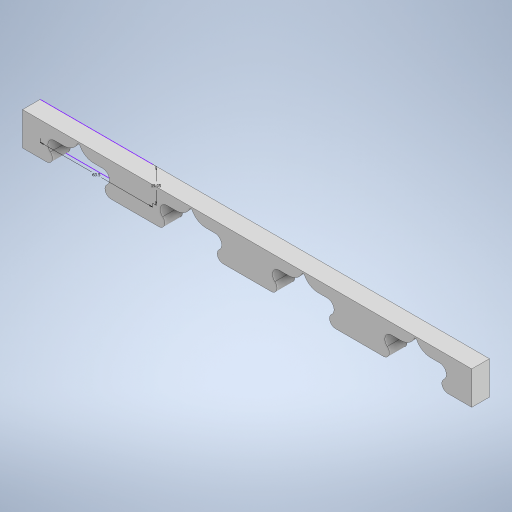
# Autodesk Inventor part: Zipperteethv2
Saved by Autodesk Inventor 2023.1 (Build 271208000, 208)
## iProperties
Created: 2022-09-20
Part Number: Zipperteethv2
Material: Generic
Document SubType Name: Modeling
Designer: Grimm
Density: 1 g/cm^3
Appearance: Default
Author: Grimm
Autodesk Inventor part; units mm, degrees
ref_plane "YZ Plane" through (0, 0, 0) normal (1, 0, 0) x (0, 1, 0)
ref_plane "XZ Plane" through (0, 0, 0) normal (0, 1, 0) x (-1, 0, 0)
ref_plane "XY Plane" through (0, 0, 0) normal (0, 0, 1) x (1, 0, 0)
sketch "Sketch1" plane through (0, 0, 0) normal (0, 0, 1) x (1, 0, 0)
  line L0 (-11.2052, 4.8709) -> (52.2948, 4.8709)
  line L1 (52.2948, 4.8709) -> (52.2948, -14.1791)
  line L2 (52.2948, -14.1791) -> (-11.2052, -14.1791)
  line L3 (-11.2052, -14.1791) -> (-11.2052, 4.8709)
  point P0 (0, 0)
  dimension "d0" = 63.5
  dimension "d1" = 19.05
  constraints: 8 end point, 2 parallel, 1 horizontal, 1 perpendicular
  measures "d0" distance of L1.end L2.end
  measures "d1" distance of L0.end L1.end
extrude "Extrusion1" add sketch "Sketch1" along normal blind 10
sketch "Sketch2" plane through (0, 0, 10) normal (0, 0, 1) x (1, 0, 0)
  line L0 (52.2948, 4.8709) -> (-11.2052, 4.8709) projected
  line L1 (20.5448, 4.8709) -> (20.5448, 2.3309)
  line L2 (-11.2052, -14.1791) -> (52.2948, -14.1791) projected
  arc A0 (7.0053, -1.4791) -> (4.6698, -7.8291) centre (7.0053, -5.0836) ccw
  arc A1 (2.3343, -14.1791) -> (4.6698, -7.8291) centre (2.3343, -10.5746) ccw
  arc A2 (36.4198, -7.8291) -> (34.0843, -1.4791) centre (34.0843, -5.0836) ccw
  arc A3 (36.4198, -7.8291) -> (38.7553, -14.1791) centre (38.7553, -10.5746) ccw
  line L3 (7.0053, -1.4791) -> (34.0843, -1.4791)
  line L4 (38.7553, -14.1791) -> (2.3343, -14.1791)
  line L5 (34.0843, -5.0836) -> (38.7553, -10.5746) construction
  line L6 (2.3343, -10.5746) -> (7.0053, -5.0836) construction
  point P0 (0, 0)
  point P1 (36.4198, -7.8291)
  point P2 (20.5448, -1.4791)
  point P3 (2.3343, -14.1791)
  dimension "d4" = 2.54
  dimension "d9" = 12.7
  dimension "d10" = 31.75
  constraints: 10 end point, 10 point on circle, 6 tangent, 4 centre point, 4 midpoint, 3 equal radius, 2 horizontal, 2 point on line, 1 vertical
  measures "d4" distance of L1.start L1.end
  measures "d9" distance between parallel lines of L2 L3
  measures "d10" distance of point (36.42, -7.829) point (4.67, -7.829)
extrude "Extrusion2" cut sketch "Sketch2" against normal through all
thicken "Thicken1" operation cut thickness 0.25 both sides no extend neighbours no toward (0, 1, 0) faces at (-6.692, -14.1791, 3.3333) (5.855, -9.8017, 6.6667) (4.4548, -7.6306, 3.3333) (25.058, -1.4791, 6.6667) (35.2349, -1.6677, 3.3333) (36.5746, -13.4446, 6.6667) (43.2685, -14.1791, 3.3333)
sketch "Sketch3" plane through (0, 0, 10) normal (0, 0, 1) x (1, 0, 0)
  arc A0 (12.085, -1.2291) -> (20.0448, 3.8709) centre (12.085, 7.5326) ccw
  arc A1 (21.0448, 3.8709) -> (29.0047, -1.2291) centre (29.0047, 7.5326) ccw
  line L0 (7.0053, -1.2291) -> (34.0843, -1.2291) projected
  line L1 (20.0448, 3.8709) -> (21.0448, 3.8709)
  line L2 (52.2948, 4.8709) -> (-11.2052, 4.8709) projected
  line L3 (34.0843, -1.2291) -> (7.0053, -1.2291) projected
  line L4 (10.4504, -1.2291) -> (26.5903, -1.2291)
  line L5 (52.2948, -13.9291) -> (52.2948, 4.8709) construction
  point P0 (0, 0)
  point P1 (20.5448, 3.8709)
  dimension "d15" = 1
  dimension "d16" = 1
  dimension "d19" = 31.75
  constraints: 4 end point, 4 point on circle, 4 point on line, 2 centre point, 2 tangent, 1 equal radius, 1 horizontal, 1 midpoint
  measures "d15" distance between parallel lines of L2 L1
  measures "d16" distance of L1.start L1.end
  measures "d19" distance from line of L5 point (20.545, 3.871)
extrude "Extrusion3" cut sketch "Sketch3" against normal through all
pattern_linear "Rectangular Pattern1" count 4 spacing 63.5 along (1, 0, 0)
shell "Shell1" thickness 1 removed faces 0
body "Solid1"
